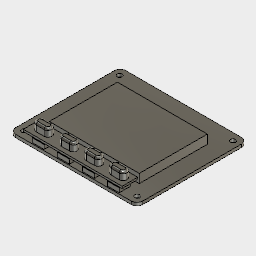
2315 PiTFT 2.2 (Autodesk Fusion 360 design; units mm, degrees)
Autodesk Fusion 360 part; units mm, degrees
sketch "pcb" plane through (0, 0, 0) normal (0, 0, 1) x (1, 0, 0)
  line L0 (0, 0) -> (65.02, 0)
  line L1 (65.02, 0) -> (65.02, -56.39)
  line L2 (65.02, -56.39) -> (0, -56.39)
  line L3 (0, -56.39) -> (0, 0)
  line L4 (32.51, -56.39) -> (32.51, 0) construction
  line L5 (0, -28.195) -> (65.02, -28.195) construction
  circle A0 centre (3.555, -3.745) radius 1.3
  circle A1 centre (61.465, -3.745) radius 1.3
  circle A2 centre (3.555, -52.645) radius 1.3
  circle A3 centre (61.465, -52.645) radius 1.3
  line L6 (10.415, -11.81) -> (56.385, -11.81)
  line L7 (56.385, -11.81) -> (56.385, -46.61)
  line L8 (56.385, -46.61) -> (10.415, -46.61)
  line L9 (10.415, -46.61) -> (10.415, -11.81)
  line L10 (33.4, -11.81) -> (33.4, -46.61) construction
  line L11 (10.415, -29.21) -> (56.385, -29.21) construction
  line L12 (55.32, -55.83) -> (49.32, -55.83)
  line L13 (49.32, -55.83) -> (49.32, -49.83)
  line L14 (49.32, -49.83) -> (55.32, -49.83)
  line L15 (55.32, -49.83) -> (55.32, -55.83)
  line L16 (55.32, -55.83) -> (49.32, -49.83) construction
  line L17 (49.32, -55.83) -> (55.32, -49.83) construction
  line L18 (36.62, -49.83) -> (42.62, -49.83)
  line L19 (36.62, -55.83) -> (36.62, -49.83)
  line L20 (42.62, -49.83) -> (42.62, -55.83)
  line L21 (42.62, -55.83) -> (36.62, -55.83)
  line L22 (23.92, -49.83) -> (29.92, -49.83)
  line L23 (23.92, -55.83) -> (23.92, -49.83)
  line L24 (29.92, -49.83) -> (29.92, -55.83)
  line L25 (29.92, -55.83) -> (23.92, -55.83)
  line L26 (16.97, -55.83) -> (10.97, -55.83)
  line L27 (10.97, -55.83) -> (10.97, -49.83)
  line L28 (10.97, -49.83) -> (16.97, -49.83)
  line L29 (16.97, -49.83) -> (16.97, -55.83)
  line L30 (16.97, -55.83) -> (10.97, -49.83) construction
  line L31 (10.97, -55.83) -> (16.97, -49.83) construction
  line L32 (26.92, -49.83) -> (26.92, -55.83) construction
  line L33 (23.92, -52.83) -> (29.92, -52.83) construction
  line L34 (39.62, -49.83) -> (39.62, -55.83) construction
  line L35 (36.62, -52.83) -> (42.62, -52.83) construction
  circle A4 centre (13.97, -52.83) radius 1.5
  circle A5 centre (26.92, -52.83) radius 1.5
  circle A6 centre (39.62, -52.83) radius 1.5
  circle A7 centre (52.32, -52.83) radius 1.5
  line L36 (7.2, -2) -> (57.82, -2)
  line L37 (57.82, -2) -> (57.82, -7)
  line L38 (57.82, -7) -> (7.2, -7)
  line L39 (7.2, -7) -> (7.2, -2)
  point P0 (52.32, -52.83)
  point P1 (13.97, -52.83)
  dimension "d1" = 65.02
  dimension "d2" = 56.39
  dimension "d3" = 2.6
  dimension "d6" = 57.91
  dimension "d7" = 48.9
  dimension "d8" = 45.97
  dimension "d9" = 34.8
  dimension "d11" = 33.4
  dimension "d12" = 27.18
  dimension "d13" = 6
  dimension "d14" = 6
  dimension "d15" = 12.7
  dimension "d16" = 3.56
  dimension "d19" = -12.7
  dimension "d20" = 0
  dimension "d21" = 6
  dimension "d22" = 6
  dimension "d24" = 3
  dimension "d25" = 3
  dimension "d26" = 3
  dimension "d27" = 3
  dimension "d28" = 50.62
  dimension "d29" = 5
  dimension "d30" = 7.2
  dimension "d31" = 2
  dimension "d80" = 13.97
  measures "d1" distance of L0.start L0.end
  measures "d2" distance of L0.start L2.end
  measures "d3" diameter of A0
  measures "d6" distance of A0.centre A1.centre
  measures "d7" distance of A0.centre A2.centre
  measures "d8" distance of L6.start L6.end
  measures "d9" distance of L6.start L8.end
  measures "d11" distance of L3 L10
  measures "d12" distance of L2 L11
  measures "d13" distance of L13.end L14.end
  measures "d14" distance of L12.end L13.end
  measures "d15" distance of L1 P0
  measures "d16" distance of L2 P0
  measures "d21" distance of L27.end L28.end
  measures "d22" distance of L26.end L27.end
  measures "d24" diameter of A4
  measures "d25" diameter of A5
  measures "d26" diameter of A6
  measures "d27" diameter of A7
  measures "d28" distance of L36.start L36.end
  measures "d29" distance of L36.start L38.end
  measures "d30" distance of L3 L39
  measures "d31" distance of L0 L36
  measures "d80" distance of L3 P1
extrude "Extrude1" add sketch "pcb" against normal blind 1.6 contours L0 L1 L2 L3 | L6 L7 L8 L9 | L12 L13 L14 L15 | L18 L19 L20 L21 | L22 L23 L24 L25 | L26 L27 L28 L29 | A4 | A5 | A6 | A7 | L36 L37 L38 L39 makes body 1
extrude "Extrude2" add sketch "pcb" along normal blind 4.5 contours L6 L7 L8 L9 bodies 1
extrude "Extrude3" add sketch "pcb" along normal blind 2.2 contours L12 L13 L14 L15 | L18 L19 L20 L21 | L22 L23 L24 L25 | L26 L27 L28 L29 | A4 | A5 | A6 | A7 bodies 1
extrude "Extrude4" add sketch "pcb" along normal blind 3.8 contours A4 | A5 | A6 | A7 bodies 1
fillet "Fillet1" radius 3 4 edges at (65.02, -56.39, -0.8) (0, 0, -0.8) (65.02, 0, -0.8) (0, -56.39, -0.8) on bodies 1
sketch "mount" plane through (0, 0, 0) normal (0, 0, 1) x (-1, 0, 0)
  arc A0 (0, 53.39) -> (-3, 56.39) centre (-3, 53.39) ccw
  line L0 (-3, 56.39) -> (-62.02, 56.39)
  arc A1 (-62.02, 56.39) -> (-65.02, 53.39) centre (-62.02, 53.39) ccw
  line L1 (-65.02, 53.39) -> (-65.02, 3)
  arc A2 (-65.02, 3) -> (-62.02, 0) centre (-62.02, 3) ccw
  line L2 (-62.02, 0) -> (-3, 0)
  arc A3 (-3, 0) -> (0, 3) centre (-3, 3) ccw
  line L3 (0, 3) -> (0, 53.39)
  line L4 (-55.32, 49.83) -> (-55.32, 55.83)
  line L5 (-55.32, 55.83) -> (-49.32, 55.83)
  line L6 (-49.32, 55.83) -> (-49.32, 49.83)
  line L7 (-49.32, 49.83) -> (-55.32, 49.83)
  line L8 (-16.97, 49.83) -> (-16.97, 55.83)
  line L9 (-16.97, 55.83) -> (-10.97, 55.83)
  line L10 (-10.97, 55.83) -> (-10.97, 49.83)
  line L11 (-10.97, 49.83) -> (-16.97, 49.83)
  line L12 (-42.62, 55.83) -> (-36.62, 55.83)
  line L13 (-36.62, 55.83) -> (-36.62, 49.83)
  line L14 (-36.62, 49.83) -> (-42.62, 49.83)
  line L15 (-42.62, 49.83) -> (-42.62, 55.83)
  line L16 (-29.92, 55.83) -> (-23.92, 55.83)
  line L17 (-23.92, 55.83) -> (-23.92, 49.83)
  line L18 (-23.92, 49.83) -> (-29.92, 49.83)
  line L19 (-29.92, 49.83) -> (-29.92, 55.83)
  line L20 (-10.415, 46.61) -> (-10.415, 11.81)
  line L21 (-10.415, 11.81) -> (-56.385, 11.81)
  line L22 (-56.385, 11.81) -> (-56.385, 46.61)
  line L23 (-56.385, 46.61) -> (-10.415, 46.61)
  circle A4 centre (-3.555, 3.745) radius 1.3
  circle A5 centre (-61.465, 3.745) radius 1.3
  circle A6 centre (-3.555, 52.645) radius 1.3
  circle A7 centre (-61.465, 52.645) radius 1.3
  circle A8 centre (-3.555, 3.745) radius 3
  circle A9 centre (-61.465, 3.745) radius 3
  circle A10 centre (-61.465, 52.645) radius 3
  circle A11 centre (-3.555, 52.645) radius 3
  dimension "d53" = 6
  dimension "d54" = 6
  dimension "d55" = 6
  dimension "d56" = 6
  measures "d53" diameter of A8
  measures "d54" diameter of A9
  measures "d55" diameter of A10
  measures "d56" diameter of A11
extrude "Extrude8" add sketch "mount" along normal blind 5.5 and the other way blind -4.5 separate body contours A0 L0 A1 L1 A2 L2 A3 L3 | L4 L5 L6 L7 | L8 L9 L10 L11 | L12 L13 L14 L15 | L16 L17 L18 L19 | A4 | A5 | A6 | A7 | A8 | A9 | A10 | A11 makes body 2
extrude "Extrude9" add sketch "mount" along normal blind 4.5 contours A4 | A5 | A6 | A7 | A8 | A9 | A10 | A11 bodies 2
extrude "Extrude10" add sketch "mount" against normal blind 3 contours A4 | A5 | A6 | A7 bodies 2
sketch "buttons" plane through (0, 0, 3.8) normal (0, 0, 1) x (-1, 0, 0)
  line L0 (-7.5, 49) -> (-58, 49)
  line L1 (-58, 49) -> (-58, 57)
  line L2 (-58, 57) -> (-7.5, 57)
  line L3 (-7.5, 57) -> (-7.5, 49)
  line L4 (-17.97, 54.83) -> (-9.97, 54.83)
  line L5 (-9.97, 54.83) -> (-9.97, 50.83)
  line L6 (-9.97, 50.83) -> (-17.97, 50.83)
  line L7 (-17.97, 50.83) -> (-17.97, 54.83)
  line L8 (-17.97, 54.83) -> (-9.97, 50.83) construction
  line L9 (-9.97, 54.83) -> (-17.97, 50.83) construction
  circle A0 centre (-26.92, 52.83) radius 1.5 construction
  circle A1 centre (-39.62, 52.83) radius 1.5 construction
  circle A2 centre (-52.32, 52.83) radius 1.5 construction
  circle A3 centre (-13.97, 52.83) radius 1.5 construction
  line L10 (-48.32, 54.83) -> (-56.32, 54.83)
  line L11 (-56.32, 54.83) -> (-56.32, 50.83)
  line L12 (-56.32, 50.83) -> (-48.32, 50.83)
  line L13 (-48.32, 50.83) -> (-48.32, 54.83)
  line L14 (-48.32, 54.83) -> (-56.32, 50.83) construction
  line L15 (-56.32, 54.83) -> (-48.32, 50.83) construction
  line L16 (-43.62, 54.83) -> (-35.62, 54.83)
  line L17 (-35.62, 54.83) -> (-35.62, 50.83)
  line L18 (-35.62, 50.83) -> (-43.62, 50.83)
  line L19 (-43.62, 50.83) -> (-43.62, 54.83)
  line L20 (-43.62, 54.83) -> (-35.62, 50.83) construction
  line L21 (-35.62, 54.83) -> (-43.62, 50.83) construction
  line L22 (-30.92, 54.83) -> (-22.92, 54.83)
  line L23 (-22.92, 54.83) -> (-22.92, 50.83)
  line L24 (-22.92, 50.83) -> (-30.92, 50.83)
  line L25 (-30.92, 50.83) -> (-30.92, 54.83)
  line L26 (-30.92, 54.83) -> (-22.92, 50.83) construction
  line L27 (-22.92, 54.83) -> (-30.92, 50.83) construction
  point P0 (-13.97, 52.83)
  point P1 (-52.32, 52.83)
  point P2 (-39.62, 52.83)
  point P3 (-26.92, 52.83)
  dimension "d66" = 8
  dimension "d67" = 4
  dimension "d68" = 8
  dimension "d69" = 4
  dimension "d70" = 8
  dimension "d71" = 4
  dimension "d72" = 8
  dimension "d73" = 4
  measures "d66" distance of L5.end L6.end
  measures "d67" distance of L4.end L5.end
  measures "d68" distance of L11.end L12.end
  measures "d69" distance of L10.end L11.end
  measures "d70" distance of L17.end L18.end
  measures "d71" distance of L16.end L17.end
  measures "d72" distance of L23.end L24.end
  measures "d73" distance of L22.end L23.end
extrude "Extrude11" add sketch "buttons" along normal blind 1 separate body contours L0 L1 L2 L3 | L4 L5 L6 L7 | L10 L11 L12 L13 | L16 L17 L18 L19 | L22 L23 L24 L25 makes body 3
extrude "Extrude12" add sketch "buttons" along normal blind 5 contours L4 L5 L6 L7 | L10 L11 L12 L13 | L16 L17 L18 L19 | L22 L23 L24 L25 bodies 3
fillet "Fillet2" radius 2 16 edges at (30.92, -50.83, 6.8) (22.92, -54.83, 6.8) (22.92, -50.83, 6.8) (48.32, -54.83, 6.8) (35.62, -54.83, 6.8) (17.97, -54.83, 6.8) (43.62, -54.83, 6.8) (56.32, -50.83, 6.8) (30.92, -54.83, 6.8) (17.97, -50.83, 6.8) (35.62, -50.83, 6.8) (48.32, -50.83, 6.8) (9.97, -50.83, 6.8) (43.62, -50.83, 6.8) (9.97, -54.83, 6.8) (56.32, -54.83, 6.8) on bodies 3
fillet "Fillet3" radius 1 16 edges at (17.97, -52.83, 8.8) (13.97, -50.83, 8.8) (9.97, -52.83, 8.8) (13.97, -54.83, 8.8) (30.92, -52.83, 8.8) (26.92, -50.83, 8.8) (22.92, -52.83, 8.8) (26.92, -54.83, 8.8) (39.62, -50.83, 8.8) (43.62, -52.83, 8.8) (39.62, -54.83, 8.8) (35.62, -52.83, 8.8) (52.32, -50.83, 8.8) (56.32, -52.83, 8.8) (52.32, -54.83, 8.8) (48.32, -52.83, 8.8) on bodies 3
hidden bodies 2
equation "d38 = 2.2 mm + 1.6 mm"
named bodies: "pitft PCB", "tester", "buttons"
